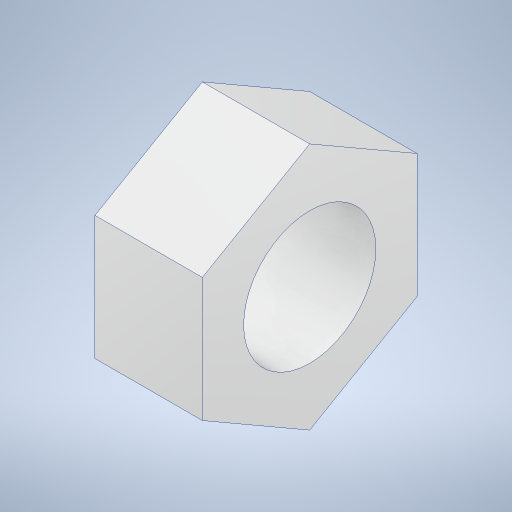
# Autodesk Inventor part: 8min-nut
Saved by Autodesk Inventor 2024.1 (Build 281209000, 209)
## iProperties
Created: 2023-11-12
Part Number: 8min-nut
Material: アルミニウム 6061
Document SubType Name: Modeling
Designer: haruy
Density: 2.7 g/cm^3
Appearance: アルミニウム - フラット
Author: haruy
Autodesk Inventor part; units mm, degrees
ref_plane "YZ Plane" through (0, 0, 0) normal (1, 0, 0) x (0, 1, 0)
ref_plane "XZ Plane" through (0, 0, 0) normal (0, 1, 0) x (-1, 0, 0)
ref_plane "XY Plane" through (0, 0, 0) normal (0, 0, 1) x (1, 0, 0)
sketch "スケッチ1" plane through (0, 0, 0) normal (1, 0, 0) x (0, 1, 0)
  circle A0 centre (0, 0) radius 7.5
  line L0 (7.5, 0) -> (3.75, 6.4952)
  line L1 (3.75, 6.4952) -> (-3.75, 6.4952)
  line L2 (-3.75, 6.4952) -> (-7.5, 0)
  line L3 (-7.5, 0) -> (-3.75, -6.4952)
  line L4 (-3.75, -6.4952) -> (3.75, -6.4952)
  line L5 (3.75, -6.4952) -> (7.5, 0)
  circle A1 centre (0, 0) radius 4
  point P0 (3.75, 6.4952)
  point P1 (-3.75, -6.4952)
  dimension "d0" = 15
  dimension "d3" = 360
  dimension "d5" = 8
  constraints: 12 end point, 3 parallel, 3 point on circle, 2 centre point, 2 coincident, 1 horizontal, 7 other
  measures "d0" diameter of A0
  measures "d5" diameter of A1
extrude "押し出し1" add sketch "スケッチ1" along normal blind 6.5 contours L5 L4 L3 L2 L1 L0
